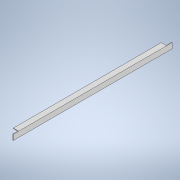
# Autodesk Inventor part: A_3030_INT
Saved by Autodesk Inventor 2020 (Build 240168000, 168)
## iProperties
Created: 2022-04-18
Part Number: A_3030_INT
Material: Genérico
Document SubType Name: Modeling
Designer: aarco
Density: 1 g/cm^3
Appearance: Valor por defecto
Author: aarco
Autodesk Inventor part; units mm, degrees
ref_plane "YZ Plane" through (0, 0, 0) normal (1, 0, 0) x (0, 1, 0)
ref_plane "XZ Plane" through (0, 0, 0) normal (0, 1, 0) x (-1, 0, 0)
ref_plane "XY Plane" through (0, 0, 0) normal (0, 0, 1) x (1, 0, 0)
sketch "Boceto1" plane through (0, 0, 0) normal (0, 1, 0) x (-1, 0, 0)
  line L0 (27, 411.5) -> (0, 411.5)
  line L1 (0, 411.5) -> (0, -411.5)
  line L2 (0, -411.5) -> (27, -411.5)
  line L3 (27, -411.5) -> (27, 411.5)
  line L4 (0, 0) -> (280.3389, 0)
  dimension "d0" = 823
  dimension "d1" = 27
  constraints: 10 end point, 2 horizontal, 2 parallel, 1 midpoint, 1 perpendicular, 1 symmetric about line
  measures "d0" distance of L2.end L0.start
  measures "d1" distance of L0.start L0.end
extrude "Extrusión1" add sketch "Boceto1" along normal blind 3
sketch "Boceto2" plane through (0, 3, 0) normal (0, 1, 0) x (1, 0, 0)
  line L0 (0, -441.5) -> (3, -441.5)
  line L1 (3, -441.5) -> (3, 441.5)
  line L2 (3, 441.5) -> (0, 441.5)
  line L3 (0, 441.5) -> (0, -441.5)
  line L4 (0, 0) -> (-318.7817, 0)
  point P0 (0, -411.5)
  dimension "d4" = 883
  dimension "d5" = 3
  constraints: 10 end point, 2 horizontal, 2 parallel, 1 perpendicular, 1 point on line, 1 symmetric about line
  measures "d4" distance of L0.end L1.end
  measures "d5" distance of L0.start L0.end
extrude "Extrusión2" add sketch "Boceto2" against normal blind 30
